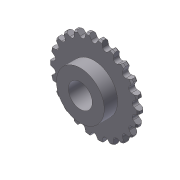
# Autodesk Inventor part: Sprocket_Num25_22T_0.5bore
Saved by Autodesk Inventor 2012 (Build 160160000, 160)
## iProperties
Created: 2012-11-22
Part Number: Sprocket_Num25_22T_0.5bore
Material: Aluminum-6061
Document SubType Name: Modeling
Designer: JesseK
Mass: 19.1782 g
Surface Area: 44.1132 cm^2
Volume: 7.07682 cm^3
Density: 2.71 g/cm^3
Author: JesseK
Autodesk Inventor part; units mm, degrees
ref_plane "YZ Plane" through (0, 0, 0) normal (1, 0, 0) x (0, 1, 0)
ref_plane "XZ Plane" through (0, 0, 0) normal (0, 1, 0) x (-1, 0, 0)
ref_plane "XY Plane" through (0, 0, 0) normal (0, 0, 1) x (1, 0, 0)
sketch "Sketch1" plane through (0, 0, 0) normal (0, 0, 1) x (1, 0, 0)
  circle A0 centre (0, 0) radius 6.35
  circle A1 centre (0, 0) radius 23.749
  dimension "d0" = 47.498
  dimension "d1" = 12.7
  constraints: 2 centre point, 2 coincident
  measures "d0" diameter of A1
  measures "d1" diameter of A0
extrude "Extrusion1" add sketch "Sketch1" along normal blind 3.1242
sketch "Sketch2" plane through (0, 0, 3.1242) normal (0, 0, 1) x (1, 0, 0)
  circle A0 centre (0, 0) radius 6.35 projected
  circle A1 centre (0, 0) radius 23.749 projected
  circle A2 centre (0, 0) radius 12.7
  circle A3 centre (0, 0) radius 6.35
  dimension "d4" = 25.4
  constraints: 2 centre point, 2 coincident, 1 concentric
  measures "d4" diameter of A2
extrude "Extrusion2" add sketch "Sketch2" along normal blind 7.1628 contours A2
sketch "Sketch3" plane through (0, 0, 0) normal (0, 0, -1) x (-1, 0, 0)
  circle A0 centre (0, 0) radius 23.749 projected
  line L0 (-2.6631, 23.5992) -> (-1.3748, 21.3678)
  line L1 (1.3748, 21.3677) -> (2.6631, 23.5992)
  arc A1 (-1.3748, 21.3678) -> (1.3748, 21.3677) centre (0, 22.1615) ccw
  circle A2 centre (0, 0) radius 22.1615 construction
  line L2 (0, 22.1615) -> (0, 0) construction
  dimension "d7" = 1.5875
  dimension "d8" = 1.5875
  dimension "d9" = 60
  constraints: 6 end point, 4 point on circle, 2 tangent, 1 centre point, 1 coincident, 1 equal length, 1 vertical, 1 vertical alignment, 2 other
  measures "d7" radius of A1
  measures "d9" angle of L1 L0
extrude "Extrusion3" cut sketch "Sketch3" against normal through all contours L1 A1 L0 A0 picked at (0.2965, 22.1559)
chamfer "Chamfer1" distance 0.7937 angle 45 2 edges at (0, -23.749, 0) (0, -23.749, 3.1242)
pattern_circular "Circular Pattern1" count 22 over 360 about axis through (0, 0, 0) along (0, 0, 1) of "Extrusion3"
body "Solid1"
